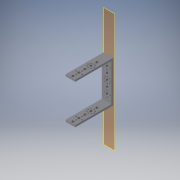
# Autodesk Inventor part: Brace
Saved by Autodesk Inventor 2016 (Build 200138000, 138)
## iProperties
Created: 2015-12-14
Part Number: Brace
Material: Generic
Document SubType Name: Modeling
Designer: Julia
Density: 1 g/cm^3
Appearance: Default
Author: Julia
Autodesk Inventor part; units mm, degrees
ref_plane "YZ Plane" through (0, 0, 0) normal (1, 0, 0) x (0, 1, 0)
ref_plane "XZ Plane" through (0, 0, 0) normal (0, 1, 0) x (-1, 0, 0)
ref_plane "XY Plane" through (0, 0, 0) normal (0, 0, 1) x (1, 0, 0)
ref_plane "Work Plane1" through (-4.081, -0.651, 0) normal (0, 0, 1) x (1, 0, 0)
sketch "Sketch1" plane through (-4.081, -0.651, 0) normal (0, 0, 1) x (1, 0, 0)
  line L0 (1.1553, -194.3642) -> (1.1553, -199.2664)
  line L1 (1.1553, -94.1016) -> (1.1553, -89.1994)
  line L2 (1.1553, -199.2664) -> (26.7608, -199.2664)
  line L3 (26.7608, -199.2664) -> (26.7608, -194.3642)
  line L4 (26.7608, -194.3642) -> (1.1553, -194.3642)
  line L5 (1.1553, -194.3642) -> (1.1553, -94.1016)
  line L6 (1.1553, -94.1016) -> (26.7608, -94.1016)
  line L7 (26.7608, -94.1016) -> (26.7608, -89.1994)
  line L8 (26.7608, -89.1994) -> (1.1553, -89.1994)
  point P0 (4.081, 0.651)
  dimension "d8" = 20.4978
  dimension "d11" = 0
  dimension "d0" = 4.9022
  dimension "d1" = 4.9022
  constraints: 18 end point, 4 perpendicular, 3 vertical, 2 horizontal
  measures "d0" distance of L0.start L0.end
  measures "d1" distance of L1.start L1.end
extrude "Extrusion1" add sketch "Sketch1" along normal blind 101.6
ref_plane "Work Plane2" through (-4.081, -0.651, 0) normal (0, 0, 1) x (1, 0, 0)
sketch "Sketch2" plane through (-4.081, -0.651, 0) normal (0, 0, 1) x (1, 0, 0)
  line L0 (1.1553, -194.3642) -> (1.1553, -199.2664) projected
  line L1 (1.1553, -94.1016) -> (26.7608, -94.1016) projected
  line L2 (1.1553, -194.3642) -> (1.1553, -94.1016)
  line L3 (1.1553, -94.1016) -> (26.7608, -94.1016)
  line L4 (26.7608, -194.3642) -> (1.1553, -194.3642) projected
  line L5 (26.7608, -94.1016) -> (26.7608, -194.3642)
  line L6 (26.7608, -194.3642) -> (1.1553, -194.3642)
  point P0 (4.081, 0.651)
  dimension "d8" = 20.4978
  dimension "d11" = 0
  constraints: 8 end point, 2 collinear, 1 perpendicular, 1 vertical
extrude "Extrusion2" add sketch "Sketch2" along normal blind 4.9022
sketch "Sketch3" plane through (-2.9257, -199.9174, 0) normal (0, -1, 0) x (1, 0, 0)
  circle A0 centre (14.8447, 24) radius 1.85 projected
  circle A1 centre (14.8447, 8) radius 1.85 projected
  circle A2 centre (6.8447, 16) radius 1.85 projected
  circle A3 centre (22.8447, 16) radius 1.85 projected
  circle A4 centre (14.8447, 16) radius 4 projected
  circle A5 centre (14.8447, 16) radius 4
  circle A6 centre (6.8447, 16) radius 1.85
  circle A7 centre (14.8447, 8) radius 1.85
  circle A8 centre (14.8447, 24) radius 1.85
  circle A9 centre (22.8447, 16) radius 1.85
  point P0 (2.9257, 0)
  constraints: 5 centre point, 5 coincident, 5 concentric
sketch "Sketch4" plane through (-2.9257, -89.8504, 0) normal (0, 1, 0) x (1, 0, 0)
  line L0 (28.3447, 32) -> (28.3447, -384) projected
  line L1 (28.3447, 32) -> (1.3447, 32) projected
  arc A0 (1.3447, 32) -> (-1.1553, 29.5) centre (1.3447, 29.5) ccw projected
  line L2 (-1.1553, -381.5) -> (-1.1553, 29.5) projected
  arc A1 (-1.1553, -381.5) -> (1.3447, -384) centre (1.3447, -381.5) ccw projected
  line L3 (28.3447, -384) -> (1.3447, -384) projected
  circle A2 centre (14.8447, -256) radius 4 projected
  circle A3 centre (14.8447, -288) radius 4 projected
  circle A4 centre (14.8447, -320) radius 4 projected
  circle A5 centre (14.8447, -352) radius 4 projected
  circle A6 centre (14.8447, 16) radius 4 projected
  circle A7 centre (6.8447, 16) radius 1.85 projected
  circle A8 centre (22.8447, 16) radius 1.85 projected
  circle A9 centre (14.8447, 8) radius 1.85 projected
  circle A10 centre (14.8447, 24) radius 1.85 projected
  circle A11 centre (9.1879, 10.3431) radius 1.85 projected
  circle A12 centre (9.1879, 21.6569) radius 1.85 projected
  circle A13 centre (20.5016, 21.6569) radius 1.85 projected
  circle A14 centre (20.5016, 10.3431) radius 1.85 projected
  circle A15 centre (14.8447, -48) radius 4 projected
  circle A16 centre (6.8447, -48) radius 1.85 projected
  circle A17 centre (22.8447, -48) radius 1.85 projected
  circle A18 centre (14.8447, -56) radius 1.85 projected
  circle A19 centre (14.8447, -40) radius 1.85 projected
  circle A20 centre (9.1879, -53.6569) radius 1.85 projected
  circle A21 centre (9.1879, -42.3431) radius 1.85 projected
  circle A22 centre (20.5016, -42.3431) radius 1.85 projected
  circle A23 centre (20.5016, -53.6569) radius 1.85 projected
  circle A24 centre (14.8447, -112) radius 4 projected
  circle A25 centre (6.8447, -112) radius 1.85 projected
  circle A26 centre (22.8447, -112) radius 1.85 projected
  circle A27 centre (14.8447, -120) radius 1.85 projected
  circle A28 centre (14.8447, -104) radius 1.85 projected
  circle A29 centre (9.1879, -117.6569) radius 1.85 projected
  circle A30 centre (9.1879, -106.3431) radius 1.85 projected
  circle A31 centre (20.5016, -106.3431) radius 1.85 projected
  circle A32 centre (20.5016, -117.6569) radius 1.85 projected
  circle A33 centre (14.8447, -176) radius 4 projected
  circle A34 centre (6.8447, -176) radius 1.85 projected
  circle A35 centre (22.8447, -176) radius 1.85 projected
  circle A36 centre (14.8447, -184) radius 1.85 projected
  circle A37 centre (14.8447, -168) radius 1.85 projected
  circle A38 centre (9.1879, -181.6569) radius 1.85 projected
  circle A39 centre (9.1879, -170.3431) radius 1.85 projected
  circle A40 centre (20.5016, -170.3431) radius 1.85 projected
  circle A41 centre (20.5016, -181.6569) radius 1.85 projected
  circle A42 centre (14.8447, -240) radius 4 projected
  circle A43 centre (6.8447, -240) radius 1.85 projected
  circle A44 centre (22.8447, -240) radius 1.85 projected
  circle A45 centre (14.8447, -248) radius 1.85 projected
  circle A46 centre (14.8447, -232) radius 1.85 projected
  circle A47 centre (9.1879, -245.6569) radius 1.85 projected
  circle A48 centre (9.1879, -234.3431) radius 1.85 projected
  circle A49 centre (20.5016, -234.3431) radius 1.85 projected
  circle A50 centre (20.5016, -245.6569) radius 1.85 projected
  circle A51 centre (14.8447, -304) radius 4 projected
  circle A52 centre (6.8447, -304) radius 1.85 projected
  circle A53 centre (22.8447, -304) radius 1.85 projected
  circle A54 centre (14.8447, -312) radius 1.85 projected
  circle A55 centre (14.8447, -296) radius 1.85 projected
  circle A56 centre (9.1879, -309.6569) radius 1.85 projected
  circle A57 centre (9.1879, -298.3431) radius 1.85 projected
  circle A58 centre (20.5016, -298.3431) radius 1.85 projected
  circle A59 centre (20.5016, -309.6569) radius 1.85 projected
  circle A60 centre (14.8447, -368) radius 4 projected
  circle A61 centre (6.8447, -368) radius 1.85 projected
  circle A62 centre (22.8447, -368) radius 1.85 projected
  circle A63 centre (14.8447, -376) radius 1.85 projected
  circle A64 centre (14.8447, -360) radius 1.85 projected
  circle A65 centre (9.1879, -373.6569) radius 1.85 projected
  circle A66 centre (9.1879, -362.3431) radius 1.85 projected
  circle A67 centre (20.5016, -362.3431) radius 1.85 projected
  circle A68 centre (20.5016, -373.6569) radius 1.85 projected
  circle A69 centre (14.8447, -16) radius 4 projected
  circle A70 centre (6.8447, -16) radius 1.85 projected
  circle A71 centre (14.8447, -24) radius 1.85 projected
  circle A72 centre (22.8447, -16) radius 1.85 projected
  circle A73 centre (14.8447, -8) radius 1.85 projected
  circle A74 centre (14.8447, -80) radius 4 projected
  circle A75 centre (6.8447, -80) radius 1.85 projected
  circle A76 centre (14.8447, -88) radius 1.85 projected
  circle A77 centre (22.8447, -80) radius 1.85 projected
  circle A78 centre (14.8447, -72) radius 1.85 projected
  circle A79 centre (14.8447, -144) radius 4 projected
  circle A80 centre (6.8447, -144) radius 1.85 projected
  circle A81 centre (14.8447, -152) radius 1.85 projected
  circle A82 centre (22.8447, -144) radius 1.85 projected
  circle A83 centre (14.8447, -136) radius 1.85 projected
  circle A84 centre (14.8447, -208) radius 4 projected
  circle A85 centre (6.8447, -208) radius 1.85 projected
  circle A86 centre (14.8447, -216) radius 1.85 projected
  circle A87 centre (22.8447, -208) radius 1.85 projected
  circle A88 centre (14.8447, -200) radius 1.85 projected
  circle A89 centre (14.8447, -272) radius 4 projected
  circle A90 centre (6.8447, -272) radius 1.85 projected
  circle A91 centre (14.8447, -280) radius 1.85 projected
  circle A92 centre (22.8447, -272) radius 1.85 projected
  circle A93 centre (14.8447, -264) radius 1.85 projected
  circle A94 centre (14.8447, -336) radius 4 projected
  circle A95 centre (6.8447, -336) radius 1.85 projected
  circle A96 centre (14.8447, -344) radius 1.85 projected
  circle A97 centre (22.8447, -336) radius 1.85 projected
  circle A98 centre (14.8447, -328) radius 1.85 projected
  circle A99 centre (14.8447, 0) radius 4 projected
  circle A100 centre (14.8447, -32) radius 4 projected
  circle A101 centre (14.8447, -64) radius 4 projected
  circle A102 centre (14.8447, -96) radius 4 projected
  circle A103 centre (14.8447, -128) radius 4 projected
  circle A104 centre (14.8447, -160) radius 4 projected
  circle A105 centre (14.8447, -192) radius 4 projected
  circle A106 centre (14.8447, -224) radius 4 projected
  circle A107 centre (14.8447, -96) radius 4
  circle A108 centre (14.8447, -88) radius 1.85
  circle A109 centre (6.8447, -80) radius 1.85
  circle A110 centre (14.8447, -80) radius 4
  circle A111 centre (22.8447, -80) radius 1.85
  circle A112 centre (14.8447, -72) radius 1.85
  circle A113 centre (14.8447, -64) radius 4
  circle A114 centre (14.8447, -56) radius 1.85
  circle A115 centre (9.1879, -53.6569) radius 1.85
  circle A116 centre (6.8447, -48) radius 1.85
  circle A117 centre (14.8447, -48) radius 4
  circle A118 centre (20.5016, -53.6569) radius 1.85
  circle A119 centre (22.8447, -48) radius 1.85
  circle A120 centre (20.5016, -42.3431) radius 1.85
  circle A121 centre (14.8447, -40) radius 1.85
  circle A122 centre (9.1879, -42.3431) radius 1.85
  circle A123 centre (14.8447, -32) radius 4
  point P0 (2.9257, 0)
  constraints: 17 centre point, 17 coincident, 17 concentric
extrude "Extrusion3" cut sketch "Sketch4" against normal blind 20.7772 contours A15 | A16 | A17 | A18 | A19 | A20 | A21 | A22 | A23 | A74 | A75 | A76 | A77 | A78 | A100 | A101 | A102
sketch "Sketch5" plane through (-4.081, -0.651, 4.9022) normal (0, 0, 1) x (1, 0, 0)
  line L0 (29.5, -0.3255) -> (29.5, -288.3255) projected
  line L1 (29.5, -0.3255) -> (2.5, -0.3255) projected
  line L2 (2.5, -0.3255) -> (2.5, -288.3255) projected
  line L3 (29.5, -288.3255) -> (2.5, -288.3255) projected
  circle A0 centre (16, -160.3255) radius 4 projected
  circle A1 centre (16, -192.3255) radius 4 projected
  circle A2 centre (16, -224.3255) radius 4 projected
  circle A3 centre (16, -256.3255) radius 4 projected
  circle A4 centre (16, -16.3255) radius 4 projected
  circle A5 centre (8, -16.3255) radius 1.85 projected
  circle A6 centre (10.3431, -21.9824) radius 1.85 projected
  circle A7 centre (16, -24.3255) radius 1.85 projected
  circle A8 centre (21.6569, -21.9824) radius 1.85 projected
  circle A9 centre (24, -16.3255) radius 1.85 projected
  circle A10 centre (21.6569, -10.6687) radius 1.85 projected
  circle A11 centre (16, -8.3255) radius 1.85 projected
  circle A12 centre (10.3431, -10.6687) radius 1.85 projected
  circle A13 centre (16, -80.3255) radius 4 projected
  circle A14 centre (8, -80.3255) radius 1.85 projected
  circle A15 centre (10.3431, -85.9824) radius 1.85 projected
  circle A16 centre (16, -88.3255) radius 1.85 projected
  circle A17 centre (21.6569, -85.9824) radius 1.85 projected
  circle A18 centre (24, -80.3255) radius 1.85 projected
  circle A19 centre (21.6569, -74.6687) radius 1.85 projected
  circle A20 centre (16, -72.3255) radius 1.85 projected
  circle A21 centre (10.3431, -74.6687) radius 1.85 projected
  circle A22 centre (16, -144.3255) radius 4 projected
  circle A23 centre (8, -144.3255) radius 1.85 projected
  circle A24 centre (10.3431, -149.9824) radius 1.85 projected
  circle A25 centre (16, -152.3255) radius 1.85 projected
  circle A26 centre (21.6569, -149.9824) radius 1.85 projected
  circle A27 centre (24, -144.3255) radius 1.85 projected
  circle A28 centre (21.6569, -138.6687) radius 1.85 projected
  circle A29 centre (16, -136.3255) radius 1.85 projected
  circle A30 centre (10.3431, -138.6687) radius 1.85 projected
  circle A31 centre (16, -208.3255) radius 4 projected
  circle A32 centre (8, -208.3255) radius 1.85 projected
  circle A33 centre (10.3431, -213.9824) radius 1.85 projected
  circle A34 centre (16, -216.3255) radius 1.85 projected
  circle A35 centre (21.6569, -213.9824) radius 1.85 projected
  circle A36 centre (24, -208.3255) radius 1.85 projected
  circle A37 centre (21.6569, -202.6687) radius 1.85 projected
  circle A38 centre (16, -200.3255) radius 1.85 projected
  circle A39 centre (10.3431, -202.6687) radius 1.85 projected
  circle A40 centre (16, -272.3255) radius 4 projected
  circle A41 centre (8, -272.3255) radius 1.85 projected
  circle A42 centre (10.3431, -277.9824) radius 1.85 projected
  circle A43 centre (16, -280.3255) radius 1.85 projected
  circle A44 centre (21.6569, -277.9824) radius 1.85 projected
  circle A45 centre (24, -272.3255) radius 1.85 projected
  circle A46 centre (21.6569, -266.6687) radius 1.85 projected
  circle A47 centre (16, -264.3255) radius 1.85 projected
  circle A48 centre (10.3431, -266.6687) radius 1.85 projected
  circle A49 centre (16, -48.3255) radius 4 projected
  circle A50 centre (8, -48.3255) radius 1.85 projected
  circle A51 centre (16, -56.3255) radius 1.85 projected
  circle A52 centre (24, -48.3255) radius 1.85 projected
  circle A53 centre (16, -40.3255) radius 1.85 projected
  circle A54 centre (16, -112.3255) radius 4 projected
  circle A55 centre (8, -112.3255) radius 1.85 projected
  circle A56 centre (16, -120.3255) radius 1.85 projected
  circle A57 centre (24, -112.3255) radius 1.85 projected
  circle A58 centre (16, -104.3255) radius 1.85 projected
  circle A59 centre (16, -176.3255) radius 4 projected
  circle A60 centre (8, -176.3255) radius 1.85 projected
  circle A61 centre (16, -184.3255) radius 1.85 projected
  circle A62 centre (24, -176.3255) radius 1.85 projected
  circle A63 centre (16, -168.3255) radius 1.85 projected
  circle A64 centre (16, -240.3255) radius 4 projected
  circle A65 centre (8, -240.3255) radius 1.85 projected
  circle A66 centre (16, -248.3255) radius 1.85 projected
  circle A67 centre (24, -240.3255) radius 1.85 projected
  circle A68 centre (16, -232.3255) radius 1.85 projected
  circle A69 centre (16, -32.3255) radius 4 projected
  circle A70 centre (16, -64.3255) radius 4 projected
  circle A71 centre (16, -96.3255) radius 4 projected
  circle A72 centre (16, -128.3255) radius 4 projected
  circle A73 centre (16, -176.3255) radius 4
  circle A74 centre (16, -184.3255) radius 1.85
  circle A75 centre (8, -176.3255) radius 1.85
  circle A76 centre (16, -168.3255) radius 1.85
  circle A77 centre (24, -176.3255) radius 1.85
  circle A78 centre (16, -160.3255) radius 4
  circle A79 centre (16, -144.3255) radius 4
  circle A80 centre (8, -144.3255) radius 1.85
  circle A81 centre (10.3431, -149.9824) radius 1.85
  circle A82 centre (16, -152.3255) radius 1.85
  circle A83 centre (21.6569, -149.9824) radius 1.85
  circle A84 centre (24, -144.3255) radius 1.85
  circle A85 centre (21.6569, -138.6687) radius 1.85
  circle A86 centre (16, -136.3255) radius 1.85
  circle A87 centre (10.3431, -138.6687) radius 1.85
  circle A88 centre (16, -128.3255) radius 4
  circle A89 centre (16, -120.3255) radius 1.85
  circle A90 centre (16, -112.3255) radius 4
  circle A91 centre (8, -112.3255) radius 1.85
  circle A92 centre (24, -112.3255) radius 1.85
  circle A93 centre (16, -104.3255) radius 1.85
  point P0 (4.081, 0.651)
  constraints: 21 centre point, 21 coincident, 21 concentric
extrude "Extrusion4" cut sketch "Sketch5" against normal blind 20.4978 contours A0 | A22 | A23 | A24 | A25 | A26 | A27 | A28 | A29 | A30 | A54 | A55 | A56 | A57 | A58 | A59 | A60 | A61 | A62 | A63 | A72
sketch "Sketch6" plane through (-2.9257, -199.9174, 0) normal (0, -1, 0) x (1, 0, 0)
  line L0 (28.3447, -32) -> (28.3447, 384) projected
  line L1 (1.3447, 384) -> (28.3447, 384) projected
  arc A0 (1.3447, 384) -> (-1.1553, 381.5) centre (1.3447, 381.5) ccw projected
  line L2 (-1.1553, 381.5) -> (-1.1553, -29.5) projected
  arc A1 (-1.1553, -29.5) -> (1.3447, -32) centre (1.3447, -29.5) ccw projected
  line L3 (1.3447, -32) -> (28.3447, -32) projected
  circle A2 centre (14.8447, 256) radius 4 projected
  circle A3 centre (14.8447, 288) radius 4 projected
  circle A4 centre (14.8447, 320) radius 4 projected
  circle A5 centre (14.8447, 352) radius 4 projected
  circle A6 centre (14.8447, -16) radius 4 projected
  circle A7 centre (6.8447, -16) radius 1.85 projected
  circle A8 centre (22.8447, -16) radius 1.85 projected
  circle A9 centre (14.8447, -8) radius 1.85 projected
  circle A10 centre (14.8447, -24) radius 1.85 projected
  circle A11 centre (9.1879, -10.3431) radius 1.85 projected
  circle A12 centre (9.1879, -21.6569) radius 1.85 projected
  circle A13 centre (20.5016, -21.6569) radius 1.85 projected
  circle A14 centre (20.5016, -10.3431) radius 1.85 projected
  circle A15 centre (14.8447, 48) radius 4 projected
  circle A16 centre (6.8447, 48) radius 1.85 projected
  circle A17 centre (22.8447, 48) radius 1.85 projected
  circle A18 centre (14.8447, 56) radius 1.85 projected
  circle A19 centre (14.8447, 40) radius 1.85 projected
  circle A20 centre (9.1879, 53.6569) radius 1.85 projected
  circle A21 centre (9.1879, 42.3431) radius 1.85 projected
  circle A22 centre (20.5016, 42.3431) radius 1.85 projected
  circle A23 centre (20.5016, 53.6569) radius 1.85 projected
  circle A24 centre (14.8447, 112) radius 4 projected
  circle A25 centre (6.8447, 112) radius 1.85 projected
  circle A26 centre (22.8447, 112) radius 1.85 projected
  circle A27 centre (14.8447, 120) radius 1.85 projected
  circle A28 centre (14.8447, 104) radius 1.85 projected
  circle A29 centre (9.1879, 117.6569) radius 1.85 projected
  circle A30 centre (9.1879, 106.3431) radius 1.85 projected
  circle A31 centre (20.5016, 106.3431) radius 1.85 projected
  circle A32 centre (20.5016, 117.6569) radius 1.85 projected
  circle A33 centre (14.8447, 176) radius 4 projected
  circle A34 centre (6.8447, 176) radius 1.85 projected
  circle A35 centre (22.8447, 176) radius 1.85 projected
  circle A36 centre (14.8447, 184) radius 1.85 projected
  circle A37 centre (14.8447, 168) radius 1.85 projected
  circle A38 centre (9.1879, 181.6569) radius 1.85 projected
  circle A39 centre (9.1879, 170.3431) radius 1.85 projected
  circle A40 centre (20.5016, 170.3431) radius 1.85 projected
  circle A41 centre (20.5016, 181.6569) radius 1.85 projected
  circle A42 centre (14.8447, 240) radius 4 projected
  circle A43 centre (6.8447, 240) radius 1.85 projected
  circle A44 centre (22.8447, 240) radius 1.85 projected
  circle A45 centre (14.8447, 248) radius 1.85 projected
  circle A46 centre (14.8447, 232) radius 1.85 projected
  circle A47 centre (9.1879, 245.6569) radius 1.85 projected
  circle A48 centre (9.1879, 234.3431) radius 1.85 projected
  circle A49 centre (20.5016, 234.3431) radius 1.85 projected
  circle A50 centre (20.5016, 245.6569) radius 1.85 projected
  circle A51 centre (14.8447, 304) radius 4 projected
  circle A52 centre (6.8447, 304) radius 1.85 projected
  circle A53 centre (22.8447, 304) radius 1.85 projected
  circle A54 centre (14.8447, 312) radius 1.85 projected
  circle A55 centre (14.8447, 296) radius 1.85 projected
  circle A56 centre (9.1879, 309.6569) radius 1.85 projected
  circle A57 centre (9.1879, 298.3431) radius 1.85 projected
  circle A58 centre (20.5016, 298.3431) radius 1.85 projected
  circle A59 centre (20.5016, 309.6569) radius 1.85 projected
  circle A60 centre (14.8447, 368) radius 4 projected
  circle A61 centre (6.8447, 368) radius 1.85 projected
  circle A62 centre (22.8447, 368) radius 1.85 projected
  circle A63 centre (14.8447, 376) radius 1.85 projected
  circle A64 centre (14.8447, 360) radius 1.85 projected
  circle A65 centre (9.1879, 373.6569) radius 1.85 projected
  circle A66 centre (9.1879, 362.3431) radius 1.85 projected
  circle A67 centre (20.5016, 362.3431) radius 1.85 projected
  circle A68 centre (20.5016, 373.6569) radius 1.85 projected
  circle A69 centre (14.8447, 16) radius 4 projected
  circle A70 centre (6.8447, 16) radius 1.85 projected
  circle A71 centre (14.8447, 24) radius 1.85 projected
  circle A72 centre (22.8447, 16) radius 1.85 projected
  circle A73 centre (14.8447, 8) radius 1.85 projected
  circle A74 centre (14.8447, 80) radius 4 projected
  circle A75 centre (6.8447, 80) radius 1.85 projected
  circle A76 centre (14.8447, 88) radius 1.85 projected
  circle A77 centre (22.8447, 80) radius 1.85 projected
  circle A78 centre (14.8447, 72) radius 1.85 projected
  circle A79 centre (14.8447, 144) radius 4 projected
  circle A80 centre (6.8447, 144) radius 1.85 projected
  circle A81 centre (14.8447, 152) radius 1.85 projected
  circle A82 centre (22.8447, 144) radius 1.85 projected
  circle A83 centre (14.8447, 136) radius 1.85 projected
  circle A84 centre (14.8447, 208) radius 4 projected
  circle A85 centre (6.8447, 208) radius 1.85 projected
  circle A86 centre (14.8447, 216) radius 1.85 projected
  circle A87 centre (22.8447, 208) radius 1.85 projected
  circle A88 centre (14.8447, 200) radius 1.85 projected
  circle A89 centre (14.8447, 272) radius 4 projected
  circle A90 centre (6.8447, 272) radius 1.85 projected
  circle A91 centre (14.8447, 280) radius 1.85 projected
  circle A92 centre (22.8447, 272) radius 1.85 projected
  circle A93 centre (14.8447, 264) radius 1.85 projected
  circle A94 centre (14.8447, 336) radius 4 projected
  circle A95 centre (6.8447, 336) radius 1.85 projected
  circle A96 centre (14.8447, 344) radius 1.85 projected
  circle A97 centre (22.8447, 336) radius 1.85 projected
  circle A98 centre (14.8447, 328) radius 1.85 projected
  circle A99 centre (14.8447, 0) radius 4 projected
  circle A100 centre (14.8447, 32) radius 4 projected
  circle A101 centre (14.8447, 64) radius 4 projected
  circle A102 centre (14.8447, 96) radius 4 projected
  circle A103 centre (14.8447, 128) radius 4 projected
  circle A104 centre (14.8447, 160) radius 4 projected
  circle A105 centre (14.8447, 192) radius 4 projected
  circle A106 centre (14.8447, 224) radius 4 projected
  circle A107 centre (14.8447, 32) radius 4 projected
  circle A108 centre (14.8447, 32) radius 4
  circle A109 centre (14.8447, 40) radius 1.85 projected
  circle A110 centre (14.8447, 40) radius 1.85
  circle A111 centre (9.1879, 42.3431) radius 1.85
  circle A112 centre (6.8447, 48) radius 1.85
  circle A113 centre (9.1879, 53.6569) radius 1.85 projected
  circle A114 centre (9.1879, 53.6569) radius 1.85
  circle A115 centre (14.8447, 56) radius 1.85 projected
  circle A116 centre (14.8447, 56) radius 1.85
  circle A117 centre (20.5016, 53.6569) radius 1.85
  circle A118 centre (22.8447, 48) radius 1.85 projected
  circle A119 centre (22.8447, 48) radius 1.85
  circle A120 centre (20.5016, 42.3431) radius 1.85
  circle A121 centre (14.8447, 48) radius 4
  circle A122 centre (14.8447, 64) radius 4
  circle A123 centre (14.8447, 72) radius 1.85 projected
  circle A124 centre (14.8447, 72) radius 1.85
  circle A125 centre (14.8447, 80) radius 4
  circle A126 centre (6.8447, 80) radius 1.85
  circle A127 centre (14.8447, 88) radius 1.85 projected
  circle A128 centre (14.8447, 88) radius 1.85
  circle A129 centre (22.8447, 80) radius 1.85 projected
  circle A130 centre (22.8447, 80) radius 1.85
  circle A131 centre (14.8447, 96) radius 4
  point P0 (2.9257, 0)
  constraints: 17 centre point, 17 coincident, 6 concentric
extrude "Extrusion5" cut sketch "Sketch6" against normal blind 36.6522 contours A15 | A16 | A17 | A18 | A19 | A20 | A21 | A22 | A23 | A74 | A75 | A76 | A77 | A78 | A100 | A101 | A102
body "Solid1"
